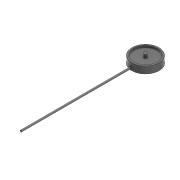
# Autodesk Inventor part: onderkant rplidar
Saved by Autodesk Inventor 2020.3 (Build 243373000, 373)
## iProperties
Created: 2020-09-30
Part Number: onderkant rplidar
Material: Acetal Resin, Black
Document SubType Name: Modeling
Designer: Svend
Density: 1.425 g/cm^3
Appearance: Smooth - Black
Author: Svend
Autodesk Inventor part; units mm, degrees
ref_plane "YZ Plane" through (0, 0, 0) normal (1, 0, 0) x (0, 1, 0)
ref_plane "XZ Plane" through (0, 0, 0) normal (0, 1, 0) x (-1, 0, 0)
ref_plane "XY Plane" through (0, 0, 0) normal (0, 0, 1) x (1, 0, 0)
sketch "Sketch1" plane through (0, 0, 0) normal (0, 0, 1) x (1, 0, 0)
  line L0 (37.85, 0) -> (37.25, 18.6)
  line L1 (37.85, 0) -> (0, 0)
  line L2 (37.25, 18.6) -> (0, 18.6)
  line L3 (0, 18.6) -> (0, 0)
  dimension "d0" = 37.85
  dimension "d1" = 37.25
  dimension "d2" = 18.6
  constraints: 8 end point, 2 horizontal, 1 vertical
  measures "d0" distance of L0.start L1.end
  measures "d1" distance of L0.end L2.end
  measures "d2" distance between parallel lines of L1 L2
revolve "Revolution1" add sketch "Sketch1" angle 360 about axis through (0, 18.6, 0) along (0, -1, 0)
sketch "Sketch2" plane through (0, 18.6, 0) normal (0, 1, 0) x (1, 0, 0)
  circle A0 centre (0, 0) radius 37.25 projected
  circle A1 centre (0, 0) radius 32.25
  point P0 (0, 0)
  dimension "d4" = 5
  constraints: 1 centre point
  measures "d4" radial gap between concentric circles of A0 A1
extrude "Extrusion1" cut sketch "Sketch2" against normal blind 5 contours A1
sketch "Sketch3" plane through (0, 13.6, 0) normal (0, 1, 0) x (1, 0, 0)
  circle A0 centre (0, 0) radius 32.25 projected
  circle A1 centre (0, 0) radius 5
  point P0 (0, 0)
  dimension "d7" = 10
  constraints: 1 centre point, 1 coincident
  measures "d7" diameter of A1
extrude "Extrusion2" add sketch "Sketch3" along normal blind 10 contours A1
fillet "Fillet1" radius 0.5 2 edges at (-37.25, 18.6, 0) (-32.25, 18.6, 0)
sketch "Sketch4" plane through (0, 0, 0) normal (1, 0, 0) x (0, 1, 0)
  line L0 (18.1161, 37.2656) -> (0, 37.85) projected
  line L1 (13.0581, 43.85) -> (5.0581, 43.85)
  line L2 (5.0581, 43.85) -> (5.0581, 37.6868)
  line L3 (0, 37.85) -> (0, -37.85) projected
  line L4 (18.1161, -37.2656) -> (18.1161, 37.2656) projected
  line L5 (13.0581, 43.85) -> (13.0581, 37.4288)
  line L6 (13.0581, 42.35) -> (12.0581, 42.35)
  line L7 (12.0581, 42.35) -> (12.0581, 41.35)
  line L8 (12.0581, 41.35) -> (13.0581, 41.35)
  line L9 (13.0581, 41.35) -> (13.0581, 42.35)
  line L10 (13.0581, 39.85) -> (12.0581, 39.85)
  line L11 (12.0581, 39.85) -> (12.0581, 38.85)
  line L12 (12.0581, 38.85) -> (13.0581, 38.85)
  line L13 (13.0581, 38.85) -> (13.0581, 39.85)
  line L14 (5.0581, 42.35) -> (6.0581, 42.35)
  line L15 (6.0581, 42.35) -> (6.0581, 41.35)
  line L16 (6.0581, 41.35) -> (5.0581, 41.35)
  line L17 (5.0581, 41.35) -> (5.0581, 42.35)
  line L18 (5.0581, 39.85) -> (6.0581, 39.85)
  line L19 (6.0581, 39.85) -> (6.0581, 38.85)
  line L20 (6.0581, 38.85) -> (5.0581, 38.85)
  line L21 (5.0581, 38.85) -> (5.0581, 39.85)
  line L22 (9.0581, 43.85) -> (9.0581, 35.85)
  line L23 (13.0581, 37.4288) -> (13.0581, 35.85)
  line L24 (13.0581, 35.85) -> (5.0581, 35.85)
  line L25 (5.0581, 35.85) -> (5.0581, 37.6868)
  point P0 (0, 0)
  point P1 (9.0581, 37.5578)
  dimension "d11" = 6
  dimension "d13" = 8
  dimension "d14" = 1
  dimension "d15" = 1.5
  dimension "d16" = 1.5
  dimension "d17" = 8
  constraints: 46 end point, 13 point on line, 9 parallel, 6 perpendicular, 5 horizontal, 4 vertical, 3 equal length, 3 midpoint, 1 vertical alignment
  measures "d11" distance from line of L0.end L1
  measures "d13" distance of L1.start L1.end
  measures "d14" distance of L6.start L6.end
  measures "d15" distance between parallel lines of L1 L14
  measures "d16" distance between parallel lines of L18 L16
  measures "d17" distance between parallel lines of L1 L24
revolve "Revolution2" add sketch "Sketch4" angle 360 about axis through (0, 9.0581, 43.85) along (0, 0, -1) contours L23 L24 L22 L0 | L0 L22 L1 L5 L6 L7 L8 L10 L11 L12
fillet "Fillet2" radius 0.3 12 edges at (3.5336, 10.9325, 37.3305) (0, 5.0581, 37.6868) (-3.5336, 10.9325, 37.3305) (0, 5.0581, 38.85) (0, 6.0581, 38.85) (0, 6.0581, 39.85) (0, 5.0581, 39.85) (0, 5.0581, 41.35) (0, 6.0581, 41.35) (0, 6.0581, 42.35) (0, 5.0581, 42.35) (0, 5.0581, 43.85)
fillet "Fillet3" radius 0.3 1 edges at (-37.85, 0, 0)
sketch "Sketch5" plane through (0, 0, 0) normal (0, -1, 0) x (1, 0, 0)
  circle A0 centre (20.75, -20.75) radius 1.5
  circle A1 centre (-20.75, -20.75) radius 1.5
  circle A2 centre (-20.75, 20.75) radius 1.5
  circle A3 centre (20.75, 20.75) radius 1.5
  line L0 (20.75, -20.75) -> (-20.75, 20.75) construction
  line L1 (-20.75, 20.75) -> (-20.75, -20.75) construction
  line L2 (-20.75, -20.75) -> (20.75, -20.75) construction
  line L3 (20.75, 20.75) -> (-20.75, -20.75) construction
  line L4 (20.75, -20.75) -> (20.75, 20.75) construction
  line L5 (-20.75, 20.75) -> (20.75, 20.75) construction
  point P0 (0, 0)
  point P1 (0, 0)
  dimension "d21" = 3
  dimension "d22" = 41.5
  constraints: 12 end point, 4 centre point, 4 perpendicular, 3 equal radius, 2 horizontal alignment, 2 vertical alignment, 1 coincident, 1 midpoint, 1 vertical
  measures "d21" diameter of A0
  measures "d22" distance of L1.end L0.start
extrude "Extrusion3" cut sketch "Sketch5" against normal blind 1
sketch "Sketch6" plane through (20.75, 1, 20.75) normal (0, -1, 0) x (1, 0, 0)
  circle A0 centre (0, 0) radius 1.5 construction
  circle A1 centre (-41.5, 0) radius 1.5 construction
  circle A2 centre (-41.5, -41.5) radius 1.5 construction
  circle A3 centre (0, -41.5) radius 1.5 construction
  point P0 (-20.75, -20.75)
  constraints: 4 coincident
hole "Hole1" at (20.75, 1, 20.75) at (-20.75, 1, 20.75) at (-20.75, 1, -20.75) at (20.75, 1, -20.75) direction (0, 1, 0) diameter 2.459 depth 8.8 tip angle 90 thread size "M3x0.5" class "6H" standard "ISO Metric profile"
sketch "Sketch7" plane through (0, 9.0581, 43.85) normal (0, 0, 1) x (1, 0, 0)
  circle A0 centre (0, 0) radius 2.75
  point P0 (0, -9.0581)
  dimension "d32" = 5.5
  constraints: 1 centre point
  measures "d32" diameter of A0
extrude "Extrusion4" add sketch "Sketch7" along normal blind 300
fillet "Fillet4" radius 1 1 edges at (-2.75, 9.0581, 343.85)
equation "\"d16\" = d15"
body "Solid1"
